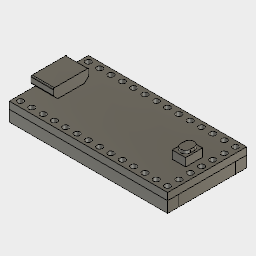
2756 Teensy 3.2 (Autodesk Fusion 360 design; units mm, degrees)
Autodesk Fusion 360 part; units mm, degrees
sketch "PCB" plane through (0, 0, 0) normal (0, 0, 1) x (1, 0, 0)
  line L0 (0, 0) -> (35.56, 0)
  line L1 (35.56, 0) -> (35.56, 17.78)
  line L2 (35.56, 17.78) -> (0, 17.78)
  line L3 (0, 17.78) -> (0, 0)
  circle A0 centre (1.27, 16.51) radius 0.65
  line L4 (0, 8.89) -> (35.56, 8.89) construction
  circle A1 centre (1.27, 1.27) radius 0.65
  circle A2 centre (3.81, 16.51) radius 0.65
  circle A3 centre (3.81, 1.27) radius 0.65
  circle A4 centre (6.35, 16.51) radius 0.65
  circle A5 centre (6.35, 1.27) radius 0.65
  circle A6 centre (8.89, 16.51) radius 0.65
  circle A7 centre (8.89, 1.27) radius 0.65
  circle A8 centre (11.43, 16.51) radius 0.65
  circle A9 centre (11.43, 1.27) radius 0.65
  circle A10 centre (13.97, 16.51) radius 0.65
  circle A11 centre (13.97, 1.27) radius 0.65
  circle A12 centre (16.51, 16.51) radius 0.65
  circle A13 centre (16.51, 1.27) radius 0.65
  circle A14 centre (19.05, 16.51) radius 0.65
  circle A15 centre (19.05, 1.27) radius 0.65
  circle A16 centre (21.59, 16.51) radius 0.65
  circle A17 centre (21.59, 1.27) radius 0.65
  circle A18 centre (24.13, 16.51) radius 0.65
  circle A19 centre (24.13, 1.27) radius 0.65
  circle A20 centre (26.67, 16.51) radius 0.65
  circle A21 centre (26.67, 1.27) radius 0.65
  circle A22 centre (29.21, 16.51) radius 0.65
  circle A23 centre (29.21, 1.27) radius 0.65
  circle A24 centre (31.75, 16.51) radius 0.65
  circle A25 centre (31.75, 1.27) radius 0.65
  circle A26 centre (34.29, 16.51) radius 0.65
  circle A27 centre (34.29, 1.27) radius 0.65
  circle A28 centre (34.29, 13.97) radius 0.65
  circle A29 centre (34.29, 11.43) radius 0.65
  circle A30 centre (34.29, 8.89) radius 0.65
  circle A31 centre (34.29, 6.35) radius 0.65
  circle A32 centre (34.29, 3.81) radius 0.65
  dimension "d1" = 35.56
  dimension "d2" = 17.78
  dimension "d5" = 1.3
  dimension "d6" = 1.27
  dimension "d7" = 1.27
  dimension "d10" = 2.54
  dimension "d11" = 0
  dimension "d12" = 1.3
  dimension "d13" = 2.54
  dimension "d16" = 0
  dimension "d17" = -2.54
  measures "d1" distance of L0.start L0.end
  measures "d2" distance of L0.start L2.end
  measures "d5" diameter of A0
  measures "d6" distance of L3 A0.centre
  measures "d7" distance of L2 A0.centre
  measures "d12" diameter of A28
  measures "d13" distance of A26.centre A28.centre
extrude "Extrude1" add sketch "PCB" along normal blind 1.6 makes body 1
sketch "USB" plane through (0, 0, 1.6) normal (0, 0, 1) x (-1, 0, 0)
  circle A0 centre (-16.51, -1.27) radius 0.65
  circle A1 centre (-1.27, -1.27) radius 0.65
  circle A2 centre (-11.43, -1.27) radius 0.65
  circle A3 centre (-29.21, -1.27) radius 0.65
  circle A4 centre (-13.97, -1.27) radius 0.65
  circle A5 centre (-21.59, -16.51) radius 0.65
  circle A6 centre (-3.81, -1.27) radius 0.65
  circle A7 centre (-26.67, -16.51) radius 0.65
  circle A8 centre (-34.29, -11.43) radius 0.65
  circle A9 centre (-8.89, -1.27) radius 0.65
  circle A10 centre (-13.97, -16.51) radius 0.65
  circle A11 centre (-16.51, -16.51) radius 0.65
  circle A12 centre (-19.05, -16.51) radius 0.65
  circle A13 centre (-34.29, -3.81) radius 0.65
  circle A14 centre (-34.29, -13.97) radius 0.65
  circle A15 centre (-29.21, -16.51) radius 0.65
  circle A16 centre (-1.27, -16.51) radius 0.65
  circle A17 centre (-26.67, -1.27) radius 0.65
  circle A18 centre (-24.13, -1.27) radius 0.65
  circle A19 centre (-24.13, -16.51) radius 0.65
  circle A20 centre (-6.35, -16.51) radius 0.65
  circle A21 centre (-3.81, -16.51) radius 0.65
  circle A22 centre (-34.29, -6.35) radius 0.65
  circle A23 centre (-11.43, -16.51) radius 0.65
  circle A24 centre (-31.75, -1.27) radius 0.65
  circle A25 centre (-19.05, -1.27) radius 0.65
  circle A26 centre (-8.89, -16.51) radius 0.65
  circle A27 centre (-6.35, -1.27) radius 0.65
  circle A28 centre (-31.75, -16.51) radius 0.65
  circle A29 centre (-21.59, -1.27) radius 0.65
  circle A30 centre (-34.29, -8.89) radius 0.65
  circle A31 centre (-34.29, -1.27) radius 0.65
  circle A32 centre (-34.29, -16.51) radius 0.65
  line L0 (0, -17.78) -> (0, 0)
  line L1 (0, 0) -> (-35.56, 0)
  line L2 (-35.56, 0) -> (-35.56, -17.78)
  line L3 (-35.56, -17.78) -> (0, -17.78)
  line L4 (0, -8.89) -> (-35.56, -8.89) construction
  line L5 (0, -12.89) -> (-5, -12.89)
  line L6 (-5, -12.89) -> (-5, -4.89)
  line L7 (-5, -4.89) -> (0, -4.89)
  line L8 (0, -4.89) -> (0, -12.89)
  line L9 (0, -8.89) -> (-5, -8.89) construction
  dimension "d18" = 5
  dimension "d19" = 8
  measures "d18" distance of L5.start L5.end
  measures "d19" distance of L5.start L7.end
extrude "Extrude2" add sketch "USB" along normal blind 2.5 separate body contours L0 L5 L6 L7 L8 makes body 2
sketch "reset" plane through (0, 0, 1.6) normal (0, 0, 1) x (-1, 0, 0)
  circle A0 centre (-16.51, -1.27) radius 0.65
  circle A1 centre (-1.27, -1.27) radius 0.65
  circle A2 centre (-11.43, -1.27) radius 0.65
  circle A3 centre (-29.21, -1.27) radius 0.65
  circle A4 centre (-13.97, -1.27) radius 0.65
  circle A5 centre (-21.59, -16.51) radius 0.65
  circle A6 centre (-3.81, -1.27) radius 0.65
  circle A7 centre (-26.67, -16.51) radius 0.65
  circle A8 centre (-34.29, -11.43) radius 0.65
  circle A9 centre (-8.89, -1.27) radius 0.65
  circle A10 centre (-13.97, -16.51) radius 0.65
  circle A11 centre (-16.51, -16.51) radius 0.65
  circle A12 centre (-19.05, -16.51) radius 0.65
  circle A13 centre (-34.29, -3.81) radius 0.65
  circle A14 centre (-34.29, -13.97) radius 0.65
  circle A15 centre (-29.21, -16.51) radius 0.65
  circle A16 centre (-1.27, -16.51) radius 0.65
  circle A17 centre (-26.67, -1.27) radius 0.65
  circle A18 centre (-24.13, -1.27) radius 0.65
  circle A19 centre (-24.13, -16.51) radius 0.65
  circle A20 centre (-6.35, -16.51) radius 0.65
  circle A21 centre (-3.81, -16.51) radius 0.65
  circle A22 centre (-34.29, -6.35) radius 0.65
  circle A23 centre (-11.43, -16.51) radius 0.65
  circle A24 centre (-31.75, -1.27) radius 0.65
  circle A25 centre (-19.05, -1.27) radius 0.65
  circle A26 centre (-8.89, -16.51) radius 0.65
  circle A27 centre (-6.35, -1.27) radius 0.65
  circle A28 centre (-31.75, -16.51) radius 0.65
  circle A29 centre (-21.59, -1.27) radius 0.65
  circle A30 centre (-34.29, -8.89) radius 0.65
  circle A31 centre (-34.29, -1.27) radius 0.65
  circle A32 centre (-34.29, -16.51) radius 0.65
  line L0 (0, -17.78) -> (0, 0)
  line L1 (0, 0) -> (-35.56, 0)
  line L2 (-35.56, 0) -> (-35.56, -17.78)
  line L3 (-35.56, -17.78) -> (0, -17.78)
  line L4 (-29.62, -10.79) -> (-32.62, -10.79)
  line L5 (-32.62, -10.79) -> (-32.62, -6.99)
  line L6 (-32.62, -6.99) -> (-29.62, -6.99)
  line L7 (-29.62, -6.99) -> (-29.62, -10.79)
  line L8 (-31.12, -10.79) -> (-31.12, -6.99) construction
  line L9 (-29.62, -8.89) -> (-32.62, -8.89) construction
  line L10 (-35.56, -8.89) -> (0, -8.89) construction
  line L11 (-30.02, -10.39) -> (-32.22, -10.39)
  line L12 (-32.22, -10.39) -> (-32.22, -7.39)
  line L13 (-32.22, -7.39) -> (-30.02, -7.39)
  line L14 (-30.02, -7.39) -> (-30.02, -10.39)
  line L15 (-30.02, -10.39) -> (-32.22, -7.39) construction
  line L16 (-32.22, -10.39) -> (-30.02, -7.39) construction
  point P0 (-31.12, -8.89)
  dimension "d22" = 3
  dimension "d23" = 3.8
  dimension "d34" = 2.2
  dimension "d35" = 3
  measures "d22" distance of L4.start L4.end
  measures "d23" distance of L4.start L6.end
  measures "d34" distance of L12.end L13.end
  measures "d35" distance of L11.end L12.end
extrude "Extrude3" add sketch "reset" along normal blind 1.8 separate body contours L4 L5 L6 L7 | L11 L12 L13 L14 makes body 3
extrude "Extrude4" add sketch "reset" along normal blind 0.7 from surface at 1.8 contours L11 L12 L13 L14 bodies 3
chamfer "Chamfer1" distance 1 angle 45 2 edges at (2.5, 12.89, 1.6) (2.5, 4.89, 1.6) on bodies 2
fillet "Fillet1" radius 0.25 6 edges at (2.5, 12.89, 4.1) (2.5, 12.89, 2.6) (2.5, 11.89, 1.6) (2.5, 4.89, 4.1) (2.5, 4.89, 2.6) (2.5, 5.89, 1.6) on bodies 2
shell "Shell1" thickness 0.4 removed faces 1 at (0, 7.9245, 3.2667) on bodies 2
fillet "Fillet2" radius 1.1 4 edges at (32.22, 10.39, 3.75) (30.02, 10.39, 3.75) (32.22, 7.39, 3.75) (30.02, 7.39, 3.75) on bodies 3
sketch "header pins" plane through (0, 0, 0) normal (0, 0, -1) x (1, 0, 0)
  circle A0 centre (16.51, -1.27) radius 0.65
  circle A1 centre (1.27, -1.27) radius 0.65
  circle A2 centre (11.43, -1.27) radius 0.65
  circle A3 centre (29.21, -1.27) radius 0.65
  circle A4 centre (13.97, -1.27) radius 0.65
  circle A5 centre (21.59, -16.51) radius 0.65
  circle A6 centre (3.81, -1.27) radius 0.65
  circle A7 centre (26.67, -16.51) radius 0.65
  circle A8 centre (34.29, -11.43) radius 0.65
  circle A9 centre (8.89, -1.27) radius 0.65
  circle A10 centre (13.97, -16.51) radius 0.65
  circle A11 centre (16.51, -16.51) radius 0.65
  circle A12 centre (19.05, -16.51) radius 0.65
  circle A13 centre (34.29, -3.81) radius 0.65
  circle A14 centre (34.29, -13.97) radius 0.65
  circle A15 centre (29.21, -16.51) radius 0.65
  circle A16 centre (1.27, -16.51) radius 0.65
  circle A17 centre (26.67, -1.27) radius 0.65
  circle A18 centre (24.13, -1.27) radius 0.65
  circle A19 centre (24.13, -16.51) radius 0.65
  circle A20 centre (6.35, -16.51) radius 0.65
  circle A21 centre (3.81, -16.51) radius 0.65
  circle A22 centre (34.29, -6.35) radius 0.65
  circle A23 centre (11.43, -16.51) radius 0.65
  circle A24 centre (31.75, -1.27) radius 0.65
  circle A25 centre (19.05, -1.27) radius 0.65
  circle A26 centre (8.89, -16.51) radius 0.65
  circle A27 centre (6.35, -1.27) radius 0.65
  circle A28 centre (31.75, -16.51) radius 0.65
  circle A29 centre (21.59, -1.27) radius 0.65
  circle A30 centre (34.29, -8.89) radius 0.65
  circle A31 centre (34.29, -1.27) radius 0.65
  circle A32 centre (34.29, -16.51) radius 0.65
  line L0 (0, 0) -> (0, -17.78)
  line L1 (0, -17.78) -> (35.56, -17.78)
  line L2 (35.56, -17.78) -> (35.56, 0)
  line L3 (35.56, 0) -> (0, 0)
  line L4 (0, 0) -> (35.56, 0)
  line L5 (35.56, 0) -> (35.56, -2.54)
  line L6 (35.56, -2.54) -> (0, -2.54)
  line L7 (0, -2.54) -> (0, 0)
  line L8 (35.56, -2.54) -> (33.02, -2.54)
  line L9 (33.02, -2.54) -> (33.02, -15.24)
  line L10 (33.02, -15.24) -> (35.56, -15.24)
  line L11 (35.56, -15.24) -> (35.56, -2.54)
  line L12 (35.56, -17.78) -> (0, -17.78)
  line L13 (0, -17.78) -> (0, -15.24)
  line L14 (0, -15.24) -> (35.56, -15.24)
  line L15 (35.56, -15.24) -> (35.56, -17.78)
  dimension "d37" = 1.27
  dimension "d38" = 1.27
  dimension "d39" = 1.27
  dimension "d40" = 1.27
  measures "d37" distance of A31.centre L6
  measures "d38" distance of A14.centre L9
  measures "d39" distance of A14.centre L10
  measures "d40" distance of A16.centre L14
extrude "Extrude5" add sketch "header pins" along normal blind 2.5 separate body contours L0 L2 L3 L4 L5 L6 L7 L8 | L0 L1 L2 L10 L12 L13 L14 L15 makes body 4 at (11.8533, 15.24, -0.8333) makes body 5 at (23.7067, 0, -0.8333)
extrude "Extrude6" add sketch "header pins" along normal blind 2.5 separate body contours L2 L6 L8 L9 L10 L11 L14 makes body 6
named bodies: "PCB", "microUSB", "reset btn"
